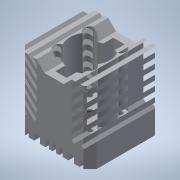
# Autodesk Inventor part: Heat Sink
Saved by Autodesk Inventor 2020 (Build 240152000, 152)
## iProperties
Created: 2012-08-27
Part Number: Heat Sink
Material: Aluminum 6061
Document SubType Name: Modeling
Designer: John
Density: 2.71 g/cm^3
Mass: 80.2934 g
Surface Area: 233.008 cm^2
Volume: 29.6286 cm^3
Appearance: Aluminum - Flat
Author: John
Autodesk Inventor part; units mm, degrees
ref_plane "YZ Plane" through (0, 0, 0) normal (1, 0, 0) x (0, 1, 0)
sketch "Sketch1" plane through (0, 0, 0) normal (0, 0, 1) x (1, 0, 0)
  line L0 (0, 0) -> (40.005, 0)
  line L1 (40.005, 0) -> (40.005, 40.005)
  line L2 (40.005, 40.005) -> (0, 40.005)
  line L3 (0, 40.005) -> (0, 0)
  dimension "d0" = 40.005
  dimension "d1" = 40.005
  constraints: 8 end point, 2 parallel, 1 horizontal, 1 perpendicular
  measures "d0" distance of L2.end L1.end
  measures "d1" distance of L1.end L0.end
extrude "Extrusion1" add sketch "Sketch1" along normal blind 40.005
sketch "Sketch2" plane through (0, 0, 0) normal (0, 0, -1) x (-1, 0, 0)
  line L0 (0, 0) -> (-40.005, 0) projected
  line L1 (0, 40.005) -> (0, 0) projected
  line L2 (-40.005, 40.005) -> (0, 40.005) projected
  line L3 (-40.005, 0) -> (-40.005, 40.005) projected
  line L4 (-3.81, 0) -> (-3.81, 40.005)
  line L5 (-5.715, 0) -> (-5.715, 40.005)
  line L6 (-8.89, 0) -> (-8.89, 40.005)
  line L7 (-12.065, 0) -> (-12.065, 40.005)
  line L8 (-15.24, 0) -> (-15.24, 40.005)
  line L9 (-17.145, 0) -> (-17.145, 40.005)
  line L10 (-19.05, 0) -> (-19.05, 40.005)
  line L11 (-20.0025, 0) -> (-20.0025, 40.005)
  line L12 (-20.955, 0) -> (-20.955, 40.005)
  line L13 (-22.86, 0) -> (-22.86, 40.005)
  line L14 (-24.765, 0) -> (-24.765, 40.005)
  line L15 (-27.94, 0) -> (-27.94, 40.005)
  line L16 (-31.115, 0) -> (-31.115, 40.005)
  line L17 (-34.29, 0) -> (-34.29, 40.005)
  line L18 (-36.195, 0) -> (-36.195, 40.005)
  dimension "d4" = 3.81
  dimension "d5" = 5.715
  dimension "d6" = 8.89
  dimension "d7" = 12.065
  dimension "d8" = 15.24
  dimension "d9" = 17.145
  dimension "d10" = 19.05
  constraints: 30 end point, 14 parallel, 39 other
  measures "d4" distance between parallel lines of L1 L4
  measures "d5" distance between parallel lines of L1 L5
  measures "d6" distance between parallel lines of L1 L6
  measures "d7" distance between parallel lines of L1 L7
  measures "d8" distance between parallel lines of L1 L8
  measures "d9" distance between parallel lines of L1 L9
  measures "d10" distance between parallel lines of L1 L10
extrude "Extrusion2" cut sketch "Sketch2" against normal blind 3.81 contours L0 L5 L2 L4 | L0 L7 L2 L6 | L0 L9 L2 L8 | L0 L11 L2 L10 | L0 L12 L2 L11 | L0 L14 L2 L13 | L0 L16 L2 L15 | L0 L18 L2 L17
sketch "Sketch3" plane through (0, 0, 0) normal (0, 0, -1) x (-1, 0, 0)
  line L0 (-3.81, 40.005) -> (-3.81, 0) projected
  line L1 (0, 0) -> (-3.81, 0) projected
  line L2 (-3.81, 40.005) -> (0, 40.005) projected
  line L3 (-36.195, 0) -> (-36.195, 40.005) projected
  line L4 (-40.005, 40.005) -> (-36.195, 40.005) projected
  line L5 (-40.005, 0) -> (-40.005, 40.005) projected
  line L6 (-36.195, 0) -> (-40.005, 0) projected
  line L7 (-36.195, 36.195) -> (-3.81, 36.195)
  line L8 (-3.81, 36.195) -> (-3.81, 3.81)
  line L9 (-3.81, 3.81) -> (-36.195, 3.81)
  line L10 (-36.195, 3.81) -> (-36.195, 36.195)
  dimension "d13" = 3.81
  dimension "d14" = 3.81
  constraints: 8 end point, 2 parallel, 2 point on line, 1 horizontal, 1 perpendicular
  measures "d13" distance between parallel lines of L2 L7
  measures "d14" distance between parallel lines of L1 L9
extrude "Extrusion3" cut sketch "Sketch3" against normal up to surface (3.81 mm away) contours L0 L9 L3 L7
sketch "Sketch4" plane through (0, 0, 3.81) normal (0, 0, -1) x (-1, 0, 0)
  line L0 (-3.81, 40.005) -> (-3.81, 0) projected
  line L1 (-36.195, 0) -> (-36.195, 40.005) projected
  line L2 (-36.195, 20.0025) -> (-3.81, 20.0025) construction
  circle A0 centre (-20.0025, 20.0025) radius 6.985
  circle A1 centre (-20.0025, 20.0025) radius 10.668
  point P0 (0, 0)
  dimension "d17" = 13.97
  dimension "d18" = 21.336
  constraints: 3 midpoint, 2 centre point, 2 end point, 1 coincident
  measures "d17" diameter of A0
  measures "d18" diameter of A1
extrude "Extrusion4" cut sketch "Sketch4" against normal blind 0.762
sketch "Sketch5" plane through (20.0025, 20.0025, 3.81) normal (0, 0, -1) x (-1, 0, 0)
  circle A0 centre (0, 0) radius 6.985 projected
  point P0 (20.0025, -20.0025)
extrude "Extrusion5" add sketch "Sketch5" along normal blind 0.508
hole "Hole1" at (20.0025, 20.0025, 3.302) direction (0, 0, 1) diameter 4.9784 end through all
sketch "Sketch6" plane through (0, 0, 3.81) normal (0, 0, -1) x (-1, 0, 0)
  circle A0 centre (-20.0025, 20.0025) radius 10.668 projected
  line L0 (-28.4861, 11.5189) -> (-11.5189, 11.5189) construction
  line L1 (-11.5189, 11.5189) -> (-11.5189, 28.4861) construction
  line L2 (-11.5189, 28.4861) -> (-28.4861, 28.4861) construction
  line L3 (-28.4861, 28.4861) -> (-28.4861, 11.5189) construction
  line L4 (-28.4861, 11.5189) -> (-11.5189, 28.4861) construction
  line L5 (-11.5189, 11.5189) -> (-28.4861, 28.4861) construction
  point P0 (0, 0)
  dimension "d32" = 16.9672
  constraints: 12 end point, 2 midpoint, 2 parallel, 2 perpendicular, 1 horizontal
  measures "d32" distance of L2.end L1.end
hole "Hole2" at (11.5189, 28.4861, 3.81) at (11.5189, 11.5189, 3.81) at (28.4861, 11.5189, 3.81) at (28.4861, 28.4861, 3.81) direction (0, 0, 1) diameter 2.667 end through all
chamfer "Chamfer1" distance 3.81 angle 45 4 edges at (0, 40.005, 20.0025) (0, 0, 20.0025) (40.005, 0, 20.0025) (40.005, 40.005, 20.0025)
sketch "Sketch7" plane through (0, 0, 40.005) normal (0, 0, 1) x (1, 0, 0)
  line L0 (36.195, 40.005) -> (3.81, 40.005) projected
  circle A0 centre (20.0025, 20.0025) radius 2.4892 projected
  line L1 (14.605, 0) -> (25.4, 0)
  line L2 (25.4, 0) -> (25.4, 40.005)
  line L3 (25.4, 40.005) -> (14.605, 40.005)
  line L4 (14.605, 40.005) -> (14.605, 0)
  line L5 (14.605, 0) -> (25.4, 40.005) construction
  line L6 (25.4, 0) -> (14.605, 40.005) construction
  point P0 (0, 0)
  dimension "d43" = 10.795
  constraints: 12 end point, 2 midpoint, 2 parallel, 1 horizontal, 1 perpendicular, 1 point on line
  measures "d43" distance of L3.end L2.end
extrude "Extrusion6" cut sketch "Sketch7" against normal blind 4.445
sketch "Sketch9" plane through (5.715, 0, 0) normal (0, -1, 0) x (1, 0, 0)
  line L0 (8.89, 35.56) -> (8.89, 40.005) projected
  line L1 (-1.905, 40.005) -> (8.89, 40.005) projected
  line L2 (19.685, 40.005) -> (30.48, 40.005) projected
  line L3 (19.685, 40.005) -> (19.685, 35.56) projected
  line L4 (19.685, 35.56) -> (8.89, 35.56) projected
  line L5 (8.89, 35.56) -> (4.445, 40.005)
  line L6 (19.685, 35.56) -> (24.13, 40.005)
  line L7 (14.2875, 35.56) -> (14.2875, 31.3012)
  point P0 (-5.715, 0)
  dimension "d54" = 45
  constraints: 6 end point, 2 point on line, 1 midpoint, 1 perpendicular, 1 other
  measures "d54" angle of L5 L0
extrude "Extrusion8" cut sketch "Sketch9" against normal through all
sketch "Sketch10" plane through (0, 0, 35.56) normal (0, 0, 1) x (1, 0, 0)
  line L0 (25.4, 40.005) -> (25.4, 0) projected
  line L1 (14.605, 40.005) -> (25.4, 40.005) projected
  line L2 (14.605, 0) -> (14.605, 40.005) projected
  line L3 (16.8275, 3.81) -> (23.1775, 3.81)
  line L4 (23.1775, 3.81) -> (23.1775, 36.195)
  line L5 (23.1775, 36.195) -> (16.8275, 36.195)
  line L6 (16.8275, 36.195) -> (16.8275, 3.81)
  line L7 (16.8275, 3.81) -> (23.1775, 36.195) construction
  line L8 (23.1775, 3.81) -> (16.8275, 36.195) construction
  line L9 (25.4, 0) -> (14.605, 0) projected
  point P0 (0, 0)
  dimension "d57" = 6.35
  dimension "d58" = 3.81
  constraints: 12 end point, 2 parallel, 1 horizontal, 1 perpendicular
  measures "d57" distance of L5.end L4.end
  measures "d58" distance between parallel lines of L1 L5
extrude "Extrusion9" cut sketch "Sketch10" against normal blind 16.51 contours L6 L5 L4 L3
sketch "Sketch11" plane through (5.715, 0, 0) normal (0, -1, 0) x (1, 0, 0)
  line L0 (-1.905, 40.005) -> (4.445, 40.005) projected
  line L1 (19.685, 35.56) -> (8.89, 35.56) projected
  line L2 (-1.905, 40.005) -> (-5.715, 40.005) projected
  line L3 (-5.715, 40.005) -> (-5.715, 0) projected
  line L4 (-5.715, 40.005) -> (4.5594, 29.7306)
  line L5 (14.2875, 35.56) -> (14.2875, 43.4297)
  line L6 (-3.0209, 40.005) -> (4.5594, 32.4247)
  line L7 (-0.3268, 40.005) -> (4.5594, 35.1187)
  line L8 (-5.715, 37.3109) -> (4.5594, 27.0365)
  line L9 (4.5594, 37.8128) -> (2.3672, 40.005)
  line L10 (4.5594, 24.3424) -> (-5.715, 34.6168)
  line L11 (4.5594, 21.6483) -> (-5.715, 31.9228)
  line L12 (4.5594, 18.9543) -> (-5.715, 29.2287)
  line L13 (4.5594, 16.2602) -> (-5.715, 26.5346)
  line L14 (4.5594, 13.5661) -> (-5.715, 23.8405)
  line L15 (4.5594, 10.872) -> (-5.715, 21.1465)
  line L16 (3.2124, 9.525) -> (-5.715, 18.4524)
  line L17 (-0.8287, 10.872) -> (-5.715, 15.7583)
  line L18 (-2.1758, 9.525) -> (-5.715, 13.0642)
  line L19 (-2.1758, 9.525) -> (-0.8287, 10.872)
  line L20 (8.89, 35.56) -> (4.445, 40.005) projected
  line L21 (30.48, 40.005) -> (30.48, 3.81) projected
  line L22 (3.2124, 9.525) -> (-5.715, 9.525)
  line L23 (3.2124, 9.525) -> (4.5594, 10.872)
  line L24 (4.5594, 10.872) -> (4.5594, 39.8906)
  point P0 (30.48, 3.81)
  dimension "d87" = 10.2744
  dimension "d61" = 45
  dimension "d66" = 1.905
  dimension "d67" = 3.81
  dimension "d73" = 1.905
  dimension "d74" = 1.905
  dimension "d75" = 1.905
  dimension "d76" = 1.905
  dimension "d77" = 1.905
  dimension "d78" = 1.905
  dimension "d79" = 1.905
  dimension "d80" = 1.905
  dimension "d81" = 1.905
  dimension "d82" = 1.905
  dimension "d83" = 1.905
  constraints: 36 end point, 12 parallel, 6 point on line, 2 horizontal, 2 perpendicular, 1 midpoint, 1 vertical, 25 other
  measures "d61" angle of L0 L4
  measures "d66" distance between parallel lines of L6 L4
  measures "d67" distance between parallel lines of L4 L7
  measures "d73" distance between parallel lines of L4 L8
  measures "d74" distance between parallel lines of L7 L9
  measures "d75" distance between parallel lines of L8 L10
  measures "d76" distance between parallel lines of L10 L11
  measures "d77" distance between parallel lines of L11 L12
  measures "d78" distance between parallel lines of L12 L13
  measures "d79" distance between parallel lines of L13 L14
  measures "d80" distance between parallel lines of L14 L15
  measures "d81" distance between parallel lines of L15 L16
  measures "d82" distance between parallel lines of L16 L17
  measures "d83" distance between parallel lines of L17 L18
extrude "Extrusion11" cut sketch "Sketch11" against normal through all contours L0 L9 L24 L7 | L6 L24 L4 L2 | L8 L24 L10 L3 | L11 L24 L12 L3 | L13 L24 L14 L3 | L15 L23 L16 L3 | L17 L19 L18 L3
ref_plane "Work Plane1" through (20.0025, 3.81, 0) normal (1, 0, 0) x (0, 0, -1)
mirror "Mirror1" about plane through (20.0025, 3.81, 0) normal (1, 0, 0) of "Extrusion11"
sketch "Sketch12" plane through (0, 0, 40.005) normal (0, 0, 1) x (1, 0, 0)
  line L0 (8.0822, 40.005) -> (8.0822, 0) projected
  line L1 (8.0822, 0) -> (10.16, 0) projected
  line L2 (10.16, 0) -> (10.16, 40.005) projected
  line L3 (10.16, 40.005) -> (8.0822, 40.005) projected
  line L4 (5.3882, 0) -> (5.3882, 40.005) projected
  line L5 (5.3882, 40.005) -> (3.81, 40.005) projected
  line L6 (2.6941, 38.8891) -> (3.81, 40.005) projected
  line L7 (2.6941, 38.8891) -> (2.6941, 1.1159) projected
  line L8 (3.81, 0) -> (2.6941, 1.1159) projected
  line L9 (3.81, 0) -> (5.3882, 0) projected
  line L10 (37.3109, 1.1159) -> (37.3109, 38.8891) projected
  line L11 (36.195, 40.005) -> (37.3109, 38.8891) projected
  line L12 (36.195, 40.005) -> (34.6168, 40.005) projected
  line L13 (34.6168, 40.005) -> (34.6168, 0) projected
  line L14 (34.6168, 0) -> (36.195, 0) projected
  line L15 (37.3109, 1.1159) -> (36.195, 0) projected
  circle A0 centre (20.0025, 20.0025) radius 2.4892 projected
  circle A1 centre (11.5189, 28.4861) radius 1.3335 projected
  circle A2 centre (11.5189, 11.5189) radius 1.3335 projected
  circle A3 centre (28.4861, 11.5189) radius 1.3335 projected
  circle A4 centre (28.4861, 28.4861) radius 1.3335 projected
  circle A5 centre (11.5189, 28.4861) radius 3.175
  circle A6 centre (11.5189, 11.5189) radius 3.175
  circle A7 centre (28.4861, 11.5189) radius 3.175
  circle A8 centre (28.4861, 28.4861) radius 3.175
  arc A9 (9.7961, 25.8191) -> (9.7961, 14.1859) centre (20.0025, 20.0025) ccw
  arc A10 (30.2089, 14.1859) -> (30.2089, 25.8191) centre (20.0025, 20.0025) ccw
  arc A11 (10.3619, 25.5294) -> (10.3619, 14.4756) centre (20.0025, 20.0025) ccw
  arc A12 (14.4756, 10.3619) -> (25.5294, 10.3619) centre (20.0025, 20.0025) ccw
  arc A13 (29.6431, 14.4756) -> (29.6431, 25.5294) centre (20.0025, 20.0025) ccw
  arc A14 (25.5294, 29.6431) -> (14.4756, 29.6431) centre (20.0025, 20.0025) ccw
  point P0 (0, 0)
  dimension "d89" = 6.35
  dimension "d91" = 11.7475
  dimension "d94" = 11.1125
  constraints: 24 point on circle, 10 centre point, 7 equal radius, 6 coincident
  measures "d89" diameter of A5
  measures "d91" radius of A9
  measures "d94" radius of A11
extrude "Extrusion12" cut sketch "Sketch12" against normal blind 31.115 contours A5 L2 | L2 A5 | A6 L2 | L2 A6 | A14 A8 A13 A7 A12 A6 A11 L2 A5 | L2 A11 | A8 | A7 | A0 | A1 | A2 | A3 | A4
extrude "Extrusion13" add sketch "Sketch12" against normal up to surface (31.115 mm away) contours A5 A11 L2 | L2 A11 A6 A9 A5 | L2 A11 A6 | A8 A10 A7 A13
sketch "Sketch13" plane through (0, 0, 0) normal (0, 0, -1) x (-1, 0, 0)
  line L0 (0, 36.195) -> (0, 3.81) projected
  line L1 (15.1172, 11.6459) -> (-3.4555, 11.6459)
  line L2 (-3.4555, 29.2227) -> (15.1172, 29.2227)
  line L3 (0, 9.1059) -> (-3.175, 9.1059)
  line L4 (-3.175, 9.1059) -> (-3.175, 31.7627)
  line L5 (-3.175, 31.7627) -> (0, 31.7627)
  line L6 (0, 31.7627) -> (0, 9.1059)
  point P0 (0, 0)
  dimension "d97" = 2.54
  dimension "d99" = 2.54
  dimension "d100" = 3.175
  constraints: 12 end point, 3 horizontal, 2 parallel, 1 perpendicular, 1 point on line, 4 other
  measures "d97" distance between parallel lines of L3 L1
  measures "d99" distance between parallel lines of L2 L5
  measures "d100" distance between parallel lines of L0 L4
ref_plane "Work Plane2" through (0, 9.1059, 0) normal (0, -1, 0) x (1, 0, 0)
sketch "Sketch14" plane through (0, 9.1059, 0) normal (0, -1, 0) x (1, 0, 0)
  line L0 (3.81, 0) -> (-1.1343, 18.4524)
  point P0 (0, 0)
  constraints: 2 end point
sweep "Sweep1" cut profiles "Sketch13" path "Sketch14"
sketch "Sketch16" plane through (0, 0, 4.572) normal (0, 0, -1) x (-1, 0, 0)
  arc A0 (-27.6134, 27.4779) -> (-27.4779, 27.6134) centre (-28.4861, 28.4861) ccw projected
  circle A1 centre (-26.3525, 27.6225) radius 0.508
  point P0 (0, 0)
  dimension "d105" = 2.1336
  dimension "d106" = 0.8636
  dimension "d107" = 1.016
  constraints: 1 centre point
  measures "d105" horizontal distance of A1.centre A0.centre
  measures "d106" vertical distance of A1.centre A0.centre
  measures "d107" diameter of A1
extrude "Extrusion14" cut sketch "Sketch16" against normal blind 0.3175
equation "\"d14\" = d13"
equation "\"d66\" = d73"
equation "\"d67\" = d65"
equation "\"d74\" = d73"
equation "\"d75\" = d73"
equation "\"d76\" = d73"
equation "\"d77\" = d73"
equation "\"d78\" = d73"
equation "\"d79\" = d73"
equation "\"d80\" = d73"
equation "\"d81\" = d73"
equation "\"d82\" = d73"
equation "\"d83\" = d73"
equation "\"d99\" = d97"
equation "\"d65\" = 3.81"
body "Solid1"
